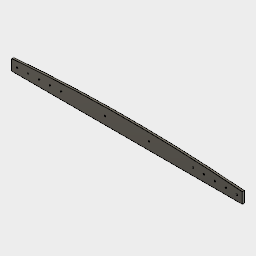
Snowboard_Mold_Basic_Public_v18 (Autodesk Fusion 360 archive; units mm, degrees)
design "Camber Block Original Public"
Autodesk Fusion 360 part; units mm, degrees
sketch "Camber Block" plane through (0, 0, 0) normal (0, 0, 1) x (1, 0, 0)
  line L0 (0, 0) -> (2133.6, 0)
  line L1 (2133.6, 0) -> (2133.6, 101.6)
  line L2 (0, 0) -> (0, 101.6)
  arc A0 (2133.6, 101.6) -> (0, 101.6) centre (1066.8, -12352.7943) ccw
  circle A1 centre (50.8, 52.9209) radius 6.35
  circle A2 centre (152.4, 56.8518) radius 6.35
  circle A3 centre (254, 60.3684) radius 6.35
  circle A4 centre (355.6, 63.4708) radius 6.35
  line L3 (1066.8, 0) -> (1066.8, 147.2057) construction
  arc A5 (2133.6, 50.8) -> (0, 50.8) centre (1066.8, -24892.1929) ccw construction
  circle A6 centre (457.2, 66.1593) radius 6.35
  circle A7 centre (863.6, 72.7759) radius 6.35
  circle A8 centre (1270, 72.7759) radius 6.35
  circle A9 centre (1676.4, 66.1593) radius 6.35
  circle A10 centre (1778, 63.4708) radius 6.35
  circle A11 centre (1879.6, 60.3684) radius 6.35
  circle A12 centre (1981.2, 56.8518) radius 6.35
  circle A13 centre (2082.8, 52.9209) radius 6.35
  line L4 (416.8, 130.2942) -> (1716.8, 130.2942) construction
  dimension "BlockWidth" = 2133.6
  dimension "EndHeight" = 101.6
  dimension "CamberRadius" = 12500
  dimension "HoleDiameter" = 12.7
  dimension "d5" = 50.8
  dimension "d7" = 101.6
  dimension "d8" = 101.6
  dimension "d9" = 101.6
  dimension "d11" = 101.6
  dimension "d12" = 406.4
  dimension "TestLine" = 1300
  dimension "d16" = 22.5203
  measures "BlockWidth" distance of L0.start L0.end
  measures "EndHeight" distance of L0.end L1.end
  measures "CamberRadius" radius of A0
  measures "HoleDiameter" diameter of A1
  measures "d5" distance of L0.start A1.centre
  measures "d7" distance of A1.centre A2.centre
  measures "d8" distance of A2.centre A3.centre
  measures "d9" distance of A3.centre A4.centre
  measures "d11" distance of A4.centre A6.centre
  measures "d12" distance of A6.centre A7.centre
  measures "TestLine" distance of L4.start L4.end
extrude "Extrude1" add sketch "Camber Block" along normal blind 19.05
equation "BlockWidth = 84\""
equation "EndHeight = 4\""
equation "d12 = 16\""
named bodies: "Camber Block Slice"

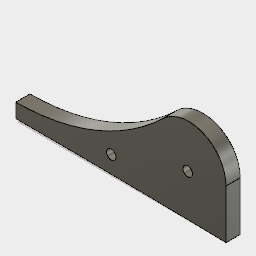
design "End Block Original #1 Public"
Autodesk Fusion 360 part; units mm, degrees
sketch "End Block Outline" plane through (0, 0, 0) normal (0, 0, 1) x (1, 0, 0)
  line L0 (0, 0) -> (0, 19.05)
  line L1 (0, 0) -> (279.4, 0) construction
  arc A0 (279.4, -3.123) -> (0, 0) centre (0, -12500) ccw
  arc A1 (0, 19.05) -> (195.4998, 97.9237) centre (0, 300.7741) ccw
  line L2 (0, 19.05) -> (279.4, 19.05) construction
  line L3 (279.4, 0) -> (279.4, -3.123) construction
  arc A2 (279.4, 62.2608) -> (195.4998, 97.9237) centre (229.8704, 62.2608) ccw
  line L4 (279.4, 62.2608) -> (279.4, -3.123)
  circle A3 centre (127, 22.225) radius 6.35
  circle A4 centre (228.6, 53.7591) radius 6.35
  line L5 (170, 19.05) -> (170, 76.1222) construction
  dimension "EndThickness" = 19.05
  dimension "BaseRadius" = 12500
  dimension "ArcRadius" = 281.7241
  dimension "BlockWidth" = 279.4
  dimension "ArcCordLength" = 210.8109
  dimension "d13" = 12.7
  dimension "d14" = 127
  dimension "d15" = 22.225
  dimension "d16" = 101.6
  dimension "d17" = 31.5341
  dimension "TestLength" = 170
  dimension "d2" = 65.002
  measures "EndThickness" distance of L0.start L0.end
  measures "BaseRadius" radius of A0
  measures "ArcRadius" radius of A1
  measures "BlockWidth" distance of L0.start L1.end
  measures "ArcCordLength" distance of L0.end A1.end
  measures "d13" diameter of A3
  measures "d14" distance of L0.end A3.centre
  measures "d15" distance of L1 A3.centre
  measures "d16" distance of A3.centre A4.centre
  measures "d17" distance of A3.centre A4.centre
  measures "TestLength" distance of L0.end L5.start
extrude "Extrude1" add sketch "End Block Outline" along normal blind 19.05
equation "BlockWidth = 11\""
equation "ArcCordLength = 2 * ArcRadius * sin(ArcAngle / 2)"
equation "d14 = 5\""
equation "d15 = ( 7 / 8 ) * 1\""
equation "d16 = 4\""
equation "ArcLength = 216.06764 mm"
equation "ArcAngle = ( 360 * ArcLength / ( 2 * PI * ArcRadius ) ) * 1 deg" comment "Internal computation"
named bodies: "End Block"
